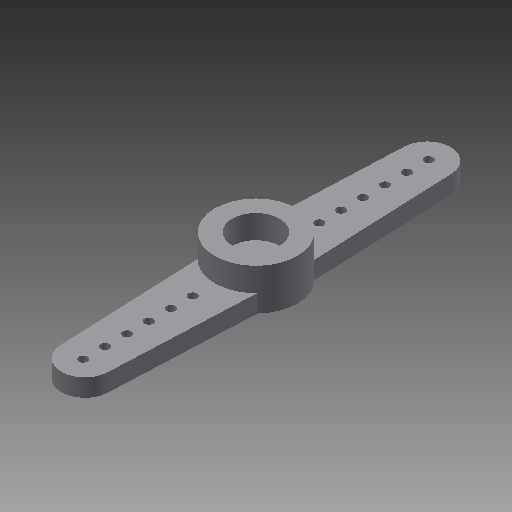
# Autodesk Inventor part: Micro Servo 9g Arm
Saved by Autodesk Inventor 2017 (Build 210142000, 142)
## iProperties
Created: 2017-03-08
Part Number: Micro Servo 9g Arm
Material: Generic
Document SubType Name: Modeling
Designer: Administrator
Density: 1 g/cm^3
Appearance: Default
Author: Administrator
Autodesk Inventor part; units mm, degrees
ref_plane "YZ Plane" through (0, 0, 0) normal (1, 0, 0) x (0, 1, 0)
ref_plane "XZ Plane" through (0, 0, 0) normal (0, 1, 0) x (-1, 0, 0)
ref_plane "XY Plane" through (0, 0, 0) normal (0, 0, 1) x (1, 0, 0)
sketch "Sketch1" plane through (0, 0, 0) normal (0, 1, 0) x (-1, 0, 0)
  line L0 (0, 0) -> (0, -16.5)
  line L1 (0, -16.5) -> (0, 16.5)
  circle A0 centre (0, -14.5) radius 2
  circle A1 centre (0, 14.5) radius 2
  line L2 (3.5, 0) -> (2.5, 0)
  line L3 (2, 14.5) -> (2.5, 2.4495)
  line L4 (2.5, -2.4495) -> (1.9983, -14.5826)
  line L5 (-1.9983, -14.5826) -> (-2.5, -2.4495)
  line L6 (-2.5299, 2.4186) -> (-1.9983, 14.5826)
  arc A2 (2.5, -2.4495) -> (2.5, 2.4495) centre (0, 0) ccw
  arc A3 (-2.5299, 2.4186) -> (-2.5, -2.4495) centre (0, 0) ccw
  dimension "d2" = 33
  dimension "d3" = 4
  dimension "d4" = 4
  dimension "d5" = 2
  dimension "d6" = 2
  dimension "d7" = 1
  constraints: 14 end point, 9 point on circle, 4 centre point, 3 point on line, 1 coincident, 1 concentric, 1 horizontal, 1 tangent, 1 vertical
  measures "d2" distance of L0.end L1.end
  measures "d3" diameter of A0
  measures "d4" diameter of A1
  measures "d5" distance of L1.end A1.centre
  measures "d6" distance of L0.end A0.centre
  measures "d7" distance of L2.start L2.end
extrude "Extrusion1" add sketch "Sketch1" along normal blind 1.5
sketch "Sketch2" plane through (0, 1.5, 0) normal (0, 1, 0) x (1, 0, 0)
  circle A0 centre (0, 0) radius 3.5
  constraints: 1 centre point, 1 coincident
extrude "Extrusion2" add sketch "Sketch2" along normal blind 2
sketch "Sketch3" plane through (0, 3.5, 0) normal (0, 1, 0) x (1, 0, 0)
  circle A0 centre (0, 0) radius 2
  dimension "d13" = 4
  constraints: 1 centre point, 1 coincident
  measures "d13" diameter of A0
extrude "Extrusion3" cut sketch "Sketch3" against normal blind 2
sketch "Sketch4" plane through (0, 1.5, 0) normal (0, 1, 0) x (1, 0, 0)
  circle A0 centre (0, 5.3571) radius 0.375
  circle A1 centre (0, 7.2143) radius 0.375
  circle A2 centre (0, 9.0714) radius 0.375
  circle A3 centre (0, 10.9286) radius 0.375
  circle A4 centre (0, 12.7857) radius 0.375
  circle A5 centre (0, 14.6429) radius 0.375
  arc A6 (2.5, 2.4495) -> (-2.5, 2.4495) centre (0, 0) ccw projected
  dimension "d16" = 0.75
  dimension "d17" = 0.75
  dimension "d18" = 0.75
  dimension "d19" = 0.75
  dimension "d20" = 0.75
  dimension "d21" = 0.75
  dimension "d22" = 1.8571
  dimension "d23" = 5.3571
  dimension "d24" = 1.8571
  dimension "d25" = 1.8571
  dimension "d26" = 1.8571
  dimension "d27" = 1.8571
  constraints: 6 centre point
  measures "d16" diameter of A0
  measures "d17" diameter of A1
  measures "d18" diameter of A2
  measures "d19" diameter of A3
  measures "d20" diameter of A4
  measures "d21" diameter of A5
  measures "d22" distance of A4.centre A5.centre
  measures "d23" distance of A0.centre A6.centre
  measures "d24" distance of A1.centre A0.centre
  measures "d25" distance of A2.centre A1.centre
  measures "d26" distance of A3.centre A2.centre
  measures "d27" distance of A4.centre A3.centre
extrude "Extrusion4" cut sketch "Sketch4" against normal blind 2
mirror "Mirror1" about plane through (0, 0, 0) normal (0, 0, 1) of "Extrusion4"
body "Solid1"
